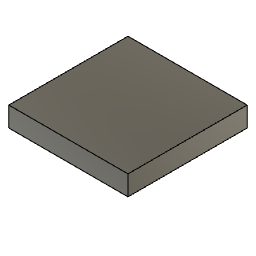
final project 3 v1 (Autodesk Fusion 360 design; units mm, degrees)
Autodesk Fusion 360 part; units mm, degrees
sketch "草图1" plane through (0, 0, 0) normal (0, 0, 1) x (1, 0, 0)
  line L0 (-9.0514, 8.5015) -> (8.9486, 8.5015)
  line L1 (8.9486, 8.5015) -> (8.9486, -9.4985)
  line L2 (8.9486, -9.4985) -> (-9.0514, -9.4985)
  line L3 (-9.0514, -9.4985) -> (-9.0514, 8.5015)
  dimension "d3" = 18
  dimension "d4" = 18
  constraint horizontal L0
  constraint vertical L1
  constraint horizontal L2
  constraint vertical L3
  measures "d3" distance of L0.start L0.end
  measures "d4" distance of L0.start L2.end
extrude "拉伸1" add sketch "草图1" along normal blind 3
sketch "草图2" plane through (0, 0, 0) normal (0, 0, 1) x (1, 0, 0)
  line L0 (-2.5482, 2.0089) -> (2.4518, 2.0089)
  line L1 (2.4518, 2.0089) -> (2.4518, -2.9911)
  line L2 (2.4518, -2.9911) -> (-2.5482, -2.9911)
  line L3 (-2.5482, -2.9911) -> (-2.5482, 2.0089)
  dimension "d7" = 5
  dimension "d8" = 5
  constraint horizontal L0
  constraint vertical L1
  constraint horizontal L2
  constraint vertical L3
  measures "d7" distance of L0.start L0.end
  measures "d8" distance of L0.start L2.end
extrude "拉伸2" add sketch "草图2" against normal blind 3
